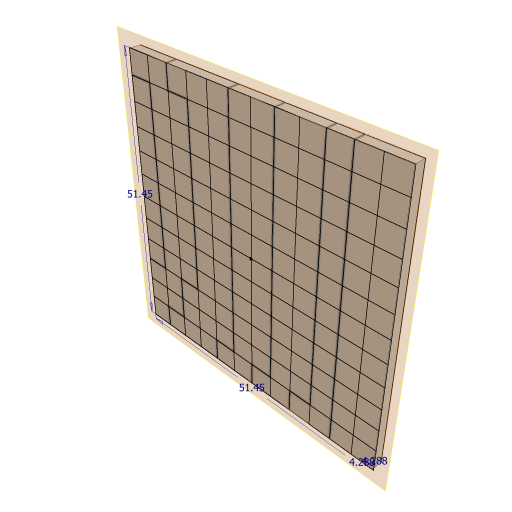
# Autodesk Inventor part: reflector_sketch
Saved by Autodesk Inventor 2023 (Build 270158000, 158)
## iProperties
Created: 2022-08-12
Part Number: reflector_sketch
Material: Generic
Document SubType Name: Modeling
Designer: James
Density: 1 g/cm^3
Appearance: Default
Author: James
Autodesk Inventor part; units mm, degrees
ref_plane "YZ Plane" through (0, 0, 0) normal (1, 0, 0) x (0, 1, 0)
ref_plane "XZ Plane" through (0, 0, 0) normal (0, 1, 0) x (-1, 0, 0)
sketch "construction_sketch" plane through (0, 0, 0) normal (0, 0, 1) x (1, 0, 0)
  line L0 (25.725, 25.725) -> (-25.725, 25.725) construction
  line L1 (-25.725, 25.725) -> (-25.725, -25.725) construction
  line L2 (-25.725, -25.725) -> (25.725, -25.725) construction
  line L3 (25.725, -25.725) -> (25.725, 25.725) construction
  line L4 (25.725, -25.725) -> (17.15, -25.725) construction
  line L5 (17.15, -25.725) -> (17.15, 25.725) construction
  line L6 (17.15, 25.725) -> (25.725, 25.725) construction
  line L7 (25.725, 25.725) -> (25.725, -25.725) construction
  line L8 (17.15, 25.725) -> (12.8625, 25.725) construction
  line L9 (12.8625, 25.725) -> (12.8625, -21.4375) construction
  line L10 (17.15, -25.725) -> (17.15, 25.725) construction
  line L11 (17.15, -25.725) -> (8.575, -25.725) construction
  line L12 (8.575, -25.725) -> (8.575, -21.4375) construction
  line L13 (8.575, -21.4375) -> (12.8625, -21.4375) construction
  line L14 (12.8625, 25.725) -> (4.2875, 25.725) construction
  line L15 (4.2875, 25.725) -> (4.2875, -21.4375) construction
  line L16 (8.575, -21.4375) -> (12.8625, -21.4375) construction
  line L17 (12.8625, -21.4375) -> (12.8625, 25.725) construction
  line L18 (8.575, -25.725) -> (0, -25.725) construction
  line L19 (0, -25.725) -> (0, -21.4375) construction
  line L20 (0, -21.4375) -> (4.2875, -21.4375) construction
  line L21 (8.575, -21.4375) -> (8.575, -25.725) construction
  line L22 (4.2875, 25.725) -> (4.2875, -21.4375) construction
  line L23 (0, -25.725) -> (0, -21.4375) construction
  line L24 (0, -21.4375) -> (4.2875, -21.4375) construction
  line L25 (4.2875, 25.725) -> (-4.2875, 25.725) construction
  line L26 (-4.2875, 25.725) -> (-4.2875, -21.4375) construction
  line L27 (0, -21.4375) -> (4.2875, -21.4375) construction
  line L28 (4.2875, -21.4375) -> (4.2875, 25.725) construction
  line L29 (0, -25.725) -> (-8.575, -25.725) construction
  line L30 (-8.575, -25.725) -> (-8.575, -21.4375) construction
  line L31 (-8.575, -21.4375) -> (-4.2875, -21.4375) construction
  line L32 (0, -21.4375) -> (0, -25.725) construction
  line L33 (-4.2875, 25.725) -> (-17.15, 25.725) construction
  line L34 (-17.15, 25.725) -> (-17.15, 21.4375) construction
  line L35 (-17.15, 21.4375) -> (-12.8625, 21.4375) construction
  line L36 (-4.2875, 21.4375) -> (-4.2875, 25.725) construction
  line L37 (-4.2875, -21.4375) -> (-8.575, -21.4375) construction
  line L38 (-17.15, -21.4375) -> (-17.15, -12.8625) construction
  line L39 (-17.15, -12.8625) -> (-12.8625, -12.8625) construction
  line L40 (-4.2875, -12.8625) -> (-4.2875, -21.4375) construction
  line L41 (-12.8625, -12.8625) -> (-12.8625, 21.4375) construction
  line L42 (-4.2875, 21.4375) -> (-4.2875, -12.8625) construction
  line L43 (-17.15, -21.4375) -> (-21.4375, -21.4375) construction
  line L44 (-21.4375, -21.4375) -> (-21.4375, -25.725) construction
  line L45 (-21.4375, -25.725) -> (-8.575, -25.725) construction
  line L46 (-8.575, -25.725) -> (-8.575, -21.4375) construction
  line L47 (-25.725, -12.8625) -> (-21.4375, -12.8625) construction
  line L48 (-21.4375, -12.8625) -> (-21.4375, 21.4375) construction
  line L49 (-21.4375, 21.4375) -> (-25.725, 21.4375) construction
  line L50 (-25.725, 21.4375) -> (-25.725, -12.8625) construction
  point P0 (0, 0)
  constraints: 102 end point, 23 parallel, 12 horizontal, 12 perpendicular, 6 point on line
sketch "construction_sketch_2" plane through (0, 0, 0) normal (0, 0, 1) x (1, 0, 0)
  line L0 (-17.15, -12.8625) -> (-12.8625, -12.8625) construction
  line L1 (25.625, 25.625) -> (25.625, -25.625) construction
  line L2 (25.625, -25.625) -> (17.25, -25.625) construction
  line L3 (17.25, -25.625) -> (17.25, 25.625) construction
  line L4 (-8.475, -25.625) -> (-8.475, -21.5375) construction
  line L5 (-8.475, -21.5375) -> (-4.1875, -21.5375) construction
  line L6 (-4.1875, -21.5375) -> (-4.1875, 25.625) construction
  line L7 (-4.1875, 25.625) -> (4.1875, 25.625) construction
  line L8 (4.1875, 25.625) -> (4.1875, -21.3375) construction
  line L9 (4.1875, -21.3375) -> (-0.1, -21.3375) construction
  line L10 (-0.1, -21.3375) -> (-0.1, -25.625) construction
  line L11 (-0.1, -25.625) -> (-8.475, -25.625) construction
  line L12 (17.25, 25.625) -> (25.625, 25.625) construction
  line L13 (4.388, 25.625) -> (12.7625, 25.625) construction
  line L14 (12.7625, 25.625) -> (12.7625, -21.3375) construction
  line L15 (12.7625, -21.3375) -> (8.475, -21.3375) construction
  line L16 (8.475, -21.3375) -> (8.475, -25.625) construction
  line L17 (8.475, -25.625) -> (0.1, -25.625) construction
  line L18 (0.1, -25.625) -> (0.1, -21.5375) construction
  line L19 (0.1, -21.5375) -> (4.388, -21.5375) construction
  line L20 (4.388, 25.625) -> (4.388, -21.5375) construction
  line L21 (17.05, -25.625) -> (17.05, 25.625) construction
  line L22 (17.05, -25.625) -> (8.675, -25.625) construction
  line L23 (8.675, -25.625) -> (8.675, -21.5375) construction
  line L24 (17.05, 25.625) -> (12.9625, 25.625) construction
  line L25 (12.9625, 25.625) -> (12.9625, -21.5375) construction
  line L26 (12.9625, -21.5375) -> (8.675, -21.5375) construction
  line L27 (-21.3375, -25.625) -> (-8.675, -25.625) construction
  line L28 (-17.0505, -21.5375) -> (-21.3375, -21.5375) construction
  line L29 (-21.3375, -21.5375) -> (-21.3375, -25.625) construction
  line L30 (-4.3875, -21.3375) -> (-8.675, -21.3375) construction
  line L31 (-4.3875, -21.3375) -> (-4.3875, 25.625) construction
  line L32 (-8.675, -25.625) -> (-8.675, -21.3375) construction
  line L33 (-4.3875, 25.625) -> (-17.0505, 25.625) construction
  line L34 (-17.0505, 25.625) -> (-17.0505, 21.537) construction
  line L35 (-17.0505, 21.537) -> (-12.7625, 21.537) construction
  line L36 (-17.0505, -21.5375) -> (-17.0505, -12.9625) construction
  line L37 (-17.0505, -12.9625) -> (-12.7625, -12.9625) construction
  line L38 (-12.7625, -12.9625) -> (-12.7625, 21.537) construction
  line L39 (-21.5375, -12.7625) -> (-25.625, -12.7625) construction
  line L40 (-25.625, -12.7625) -> (-25.625, 21.3375) construction
  line L41 (-25.625, 21.3375) -> (-21.5375, 21.3375) construction
  line L42 (-21.5375, 21.3375) -> (-21.5375, -12.7625) construction
  line L43 (-25.625, 21.5375) -> (-25.625, 25.625) construction
  line L44 (-25.625, 25.625) -> (-17.25, 25.625) construction
  line L45 (-17.25, 25.625) -> (-17.25, 21.3375) construction
  line L46 (-17.25, 21.3375) -> (-12.9625, 21.3375) construction
  line L47 (-12.9625, 21.3375) -> (-12.9625, -12.7625) construction
  line L48 (-12.9625, -12.7625) -> (-17.25, -12.7625) construction
  line L49 (-17.25, -12.7625) -> (-17.25, -21.3375) construction
  line L50 (-17.25, -21.3375) -> (-21.5375, -21.3375) construction
  line L51 (-21.5375, -21.3375) -> (-21.5375, -25.625) construction
  line L52 (-25.625, -12.9625) -> (-25.625, -25.625) construction
  line L53 (-25.625, -25.625) -> (-21.5375, -25.625) construction
  line L54 (-21.3375, -12.9625) -> (-25.625, -12.9625) construction
  line L55 (-25.625, 21.5375) -> (-21.3375, 21.5375) construction
  line L56 (-21.3375, 21.5375) -> (-21.3375, -12.9625) construction
  point P0 (0, 0)
  constraints: 114 end point, 18 perpendicular, 8 parallel, 2 horizontal, 1 point on line, 1 vertical
sketch "brick_sketch_0.1mm tolerance" plane through (0, 0, 0) normal (0, 0, 1) x (1, 0, 0)
  line L0 (-17.15, -12.8625) -> (-12.8625, -12.8625) construction
  line L1 (25.625, 25.625) -> (25.625, -25.625)
  line L2 (25.625, -25.625) -> (17.25, -25.625)
  line L3 (17.25, -25.625) -> (17.25, 25.625)
  line L4 (-8.475, -25.625) -> (-8.475, -21.5375)
  line L5 (-8.475, -21.5375) -> (-4.1875, -21.5375)
  line L6 (-4.1875, -21.5375) -> (-4.1875, 25.625)
  line L7 (-4.1875, 25.625) -> (4.1875, 25.625)
  line L8 (4.1875, 25.625) -> (4.1875, -21.3375)
  line L9 (4.1875, -21.3375) -> (-0.1, -21.3375)
  line L10 (-0.1, -21.3375) -> (-0.1, -25.625)
  line L11 (-0.1, -25.625) -> (-8.475, -25.625)
  line L12 (17.25, 25.625) -> (25.625, 25.625)
  line L13 (4.388, 25.625) -> (12.7625, 25.625)
  line L14 (12.7625, 25.625) -> (12.7625, -21.3375)
  line L15 (12.7625, -21.3375) -> (8.475, -21.3375)
  line L16 (8.475, -21.3375) -> (8.475, -25.625)
  line L17 (8.475, -25.625) -> (0.1, -25.625)
  line L18 (0.1, -25.625) -> (0.1, -21.5375)
  line L19 (0.1, -21.5375) -> (4.388, -21.5375)
  line L20 (4.388, 25.625) -> (4.388, -21.5375)
  line L21 (17.05, -25.625) -> (17.05, 25.625)
  line L22 (17.05, -25.625) -> (8.675, -25.625)
  line L23 (8.675, -25.625) -> (8.675, -21.5375)
  line L24 (17.05, 25.625) -> (12.9625, 25.625)
  line L25 (12.9625, 25.625) -> (12.9625, -21.5375)
  line L26 (12.9625, -21.5375) -> (8.675, -21.5375)
  line L27 (-21.3375, -25.625) -> (-8.675, -25.625)
  line L28 (-17.0505, -21.5375) -> (-21.3375, -21.5375)
  line L29 (-21.3375, -21.5375) -> (-21.3375, -25.625)
  line L30 (-4.3875, -21.3375) -> (-8.675, -21.3375)
  line L31 (-4.3875, -21.3375) -> (-4.3875, 25.625)
  line L32 (-8.675, -25.625) -> (-8.675, -21.3375)
  line L33 (-4.3875, 25.625) -> (-17.0505, 25.625)
  line L34 (-17.0505, 25.625) -> (-17.0505, 21.537)
  line L35 (-17.0505, 21.537) -> (-12.7625, 21.537)
  line L36 (-17.0505, -21.5375) -> (-17.0505, -12.9625)
  line L37 (-17.0505, -12.9625) -> (-12.7625, -12.9625)
  line L38 (-12.7625, -12.9625) -> (-12.7625, 21.537)
  line L39 (-21.5375, -12.7625) -> (-25.625, -12.7625)
  line L40 (-25.625, -12.7625) -> (-25.625, 21.3375)
  line L41 (-25.625, 21.3375) -> (-21.5375, 21.3375)
  line L42 (-21.5375, 21.3375) -> (-21.5375, -12.7625)
  line L43 (-25.625, 21.5375) -> (-25.625, 25.625)
  line L44 (-25.625, 25.625) -> (-17.25, 25.625)
  line L45 (-17.25, 25.625) -> (-17.25, 21.3375)
  line L46 (-17.25, 21.3375) -> (-12.9625, 21.3375)
  line L47 (-12.9625, 21.3375) -> (-12.9625, -12.7625)
  line L48 (-12.9625, -12.7625) -> (-17.25, -12.7625)
  line L49 (-17.25, -12.7625) -> (-17.25, -21.3375)
  line L50 (-17.25, -21.3375) -> (-21.5375, -21.3375)
  line L51 (-21.5375, -21.3375) -> (-21.5375, -25.625)
  line L52 (-25.625, -12.9625) -> (-25.625, -25.625)
  line L53 (-25.625, -25.625) -> (-21.5375, -25.625)
  line L54 (-21.3375, -12.9625) -> (-25.625, -12.9625)
  line L55 (-25.625, 21.5375) -> (-21.3375, 21.5375)
  line L56 (-21.3375, 21.5375) -> (-21.3375, -12.9625)
  point P0 (0, 0)
  point P1 (0, 0)
  constraints: 114 end point, 18 perpendicular, 8 parallel, 2 horizontal, 1 point on line, 1 vertical
ref_plane "Work Plane1" through (0, 0, 2) normal (0, 0, 1) x (1, 0, 0)
sketch "Sketch4" plane through (0, 0, 2) normal (0, 0, 1) x (1, 0, 0)
  line L0 (25.725, 25.725) -> (-25.725, 25.725) construction
  line L1 (-25.725, 25.725) -> (-25.725, -25.725) construction
  line L2 (-25.725, -25.725) -> (25.725, -25.725) construction
  line L3 (25.725, -25.725) -> (25.725, 25.725) construction
  line L4 (25.725, -25.725) -> (21.4375, -25.725)
  line L5 (21.4375, -25.725) -> (21.4375, -21.4375)
  line L6 (21.4375, -21.4375) -> (25.725, -21.4375)
  line L7 (25.725, -21.4375) -> (25.725, -25.725)
  line L8 (21.4375, -25.725) -> (17.15, -25.725)
  line L9 (17.15, -25.725) -> (17.15, -21.4375)
  line L10 (17.15, -21.4375) -> (21.4375, -21.4375)
  line L11 (21.4375, -21.4375) -> (21.4375, -25.725)
  line L12 (17.15, -25.725) -> (12.8625, -25.725)
  line L13 (12.8625, -25.725) -> (12.8625, -21.4375)
  line L14 (12.8625, -21.4375) -> (17.15, -21.4375)
  line L15 (17.15, -21.4375) -> (17.15, -25.725)
  line L16 (12.8625, -25.725) -> (8.575, -25.725)
  line L17 (8.575, -25.725) -> (8.575, -21.4375)
  line L18 (8.575, -21.4375) -> (12.8625, -21.4375)
  line L19 (12.8625, -21.4375) -> (12.8625, -25.725)
  line L20 (8.575, -25.725) -> (4.2875, -25.725)
  line L21 (4.2875, -25.725) -> (4.2875, -21.4375)
  line L22 (4.2875, -21.4375) -> (8.575, -21.4375)
  line L23 (8.575, -21.4375) -> (8.575, -25.725)
  line L24 (4.2875, -25.725) -> (0, -25.725)
  line L25 (0, -25.725) -> (0, -21.4375)
  line L26 (0, -21.4375) -> (4.2875, -21.4375)
  line L27 (4.2875, -21.4375) -> (4.2875, -25.725)
  line L28 (0, -25.725) -> (-4.2875, -25.725)
  line L29 (-4.2875, -25.725) -> (-4.2875, -21.4375)
  line L30 (-4.2875, -21.4375) -> (0, -21.4375)
  line L31 (0, -21.4375) -> (0, -25.725)
  line L32 (-4.2875, -25.725) -> (-8.575, -25.725)
  line L33 (-8.575, -25.725) -> (-8.575, -21.4375)
  line L34 (-8.575, -21.4375) -> (-4.2875, -21.4375)
  line L35 (-4.2875, -21.4375) -> (-4.2875, -25.725)
  line L36 (-8.575, -25.725) -> (-12.8625, -25.725)
  line L37 (-12.8625, -25.725) -> (-12.8625, -21.4375)
  line L38 (-12.8625, -21.4375) -> (-8.575, -21.4375)
  line L39 (-8.575, -21.4375) -> (-8.575, -25.725)
  line L40 (-12.8625, -25.725) -> (-17.15, -25.725)
  line L41 (-17.15, -25.725) -> (-17.15, -21.4375)
  line L42 (-17.15, -21.4375) -> (-12.8625, -21.4375)
  line L43 (-12.8625, -21.4375) -> (-12.8625, -25.725)
  line L44 (-17.15, -25.725) -> (-21.4375, -25.725)
  line L45 (-21.4375, -25.725) -> (-21.4375, -21.4375)
  line L46 (-21.4375, -21.4375) -> (-17.15, -21.4375)
  line L47 (-17.15, -21.4375) -> (-17.15, -25.725)
  line L48 (-21.4375, -25.725) -> (-25.725, -25.725)
  line L49 (-25.725, -25.725) -> (-25.725, -21.4375)
  line L50 (-25.725, -21.4375) -> (-21.4375, -21.4375)
  line L51 (-21.4375, -21.4375) -> (-21.4375, -25.725)
  line L52 (25.725, -21.4375) -> (21.4375, -21.4375)
  line L53 (21.4375, -21.4375) -> (21.4375, -17.15)
  line L54 (21.4375, -17.15) -> (25.725, -17.15)
  line L55 (25.725, -17.15) -> (25.725, -21.4375)
  line L56 (21.4375, -21.4375) -> (17.15, -21.4375)
  line L57 (17.15, -21.4375) -> (17.15, -17.15)
  line L58 (17.15, -17.15) -> (21.4375, -17.15)
  line L59 (21.4375, -17.15) -> (21.4375, -21.4375)
  line L60 (17.15, -21.4375) -> (12.8625, -21.4375)
  line L61 (12.8625, -21.4375) -> (12.8625, -17.15)
  line L62 (12.8625, -17.15) -> (17.15, -17.15)
  line L63 (17.15, -17.15) -> (17.15, -21.4375)
  line L64 (12.8625, -21.4375) -> (8.575, -21.4375)
  line L65 (8.575, -21.4375) -> (8.575, -17.15)
  line L66 (8.575, -17.15) -> (12.8625, -17.15)
  line L67 (12.8625, -17.15) -> (12.8625, -21.4375)
  line L68 (8.575, -21.4375) -> (4.2875, -21.4375)
  line L69 (4.2875, -21.4375) -> (4.2875, -17.15)
  line L70 (4.2875, -17.15) -> (8.575, -17.15)
  line L71 (8.575, -17.15) -> (8.575, -21.4375)
  line L72 (4.2875, -21.4375) -> (0, -21.4375)
  line L73 (0, -21.4375) -> (0, -17.15)
  line L74 (0, -17.15) -> (4.2875, -17.15)
  line L75 (4.2875, -17.15) -> (4.2875, -21.4375)
  line L76 (0, -21.4375) -> (-4.2875, -21.4375)
  line L77 (-4.2875, -21.4375) -> (-4.2875, -17.15)
  line L78 (-4.2875, -17.15) -> (0, -17.15)
  line L79 (0, -17.15) -> (0, -21.4375)
  line L80 (-4.2875, -21.4375) -> (-8.575, -21.4375)
  line L81 (-8.575, -21.4375) -> (-8.575, -17.15)
  line L82 (-8.575, -17.15) -> (-4.2875, -17.15)
  line L83 (-4.2875, -17.15) -> (-4.2875, -21.4375)
  line L84 (-8.575, -21.4375) -> (-12.8625, -21.4375)
  line L85 (-12.8625, -21.4375) -> (-12.8625, -17.15)
  line L86 (-12.8625, -17.15) -> (-8.575, -17.15)
  line L87 (-8.575, -17.15) -> (-8.575, -21.4375)
  line L88 (-12.8625, -21.4375) -> (-17.15, -21.4375)
  line L89 (-17.15, -21.4375) -> (-17.15, -17.15)
  line L90 (-17.15, -17.15) -> (-12.8625, -17.15)
  line L91 (-12.8625, -17.15) -> (-12.8625, -21.4375)
  line L92 (-17.15, -21.4375) -> (-21.4375, -21.4375)
  line L93 (-21.4375, -21.4375) -> (-21.4375, -17.15)
  line L94 (-21.4375, -17.15) -> (-17.15, -17.15)
  line L95 (-17.15, -17.15) -> (-17.15, -21.4375)
  line L96 (-21.4375, -21.4375) -> (-25.725, -21.4375)
  line L97 (-25.725, -21.4375) -> (-25.725, -17.15)
  line L98 (-25.725, -17.15) -> (-21.4375, -17.15)
  line L99 (-21.4375, -17.15) -> (-21.4375, -21.4375)
  line L100 (25.725, -17.15) -> (21.4375, -17.15)
  line L101 (21.4375, -17.15) -> (21.4375, -12.8625)
  line L102 (21.4375, -12.8625) -> (25.725, -12.8625)
  line L103 (25.725, -12.8625) -> (25.725, -17.15)
  line L104 (21.4375, -17.15) -> (17.15, -17.15)
  line L105 (17.15, -17.15) -> (17.15, -12.8625)
  line L106 (17.15, -12.8625) -> (21.4375, -12.8625)
  line L107 (21.4375, -12.8625) -> (21.4375, -17.15)
  line L108 (17.15, -17.15) -> (12.8625, -17.15)
  line L109 (12.8625, -17.15) -> (12.8625, -12.8625)
  line L110 (12.8625, -12.8625) -> (17.15, -12.8625)
  line L111 (17.15, -12.8625) -> (17.15, -17.15)
  line L112 (12.8625, -17.15) -> (8.575, -17.15)
  line L113 (8.575, -17.15) -> (8.575, -12.8625)
  line L114 (8.575, -12.8625) -> (12.8625, -12.8625)
  line L115 (12.8625, -12.8625) -> (12.8625, -17.15)
  line L116 (8.575, -17.15) -> (4.2875, -17.15)
  line L117 (4.2875, -17.15) -> (4.2875, -12.8625)
  line L118 (4.2875, -12.8625) -> (8.575, -12.8625)
  line L119 (8.575, -12.8625) -> (8.575, -17.15)
  line L120 (4.2875, -17.15) -> (0, -17.15)
  line L121 (0, -17.15) -> (0, -12.8625)
  line L122 (0, -12.8625) -> (4.2875, -12.8625)
  line L123 (4.2875, -12.8625) -> (4.2875, -17.15)
  line L124 (0, -17.15) -> (-4.2875, -17.15)
  line L125 (-4.2875, -17.15) -> (-4.2875, -12.8625)
  line L126 (-4.2875, -12.8625) -> (0, -12.8625)
  line L127 (0, -12.8625) -> (0, -17.15)
  line L128 (-4.2875, -17.15) -> (-8.575, -17.15)
  line L129 (-8.575, -17.15) -> (-8.575, -12.8625)
  line L130 (-8.575, -12.8625) -> (-4.2875, -12.8625)
  line L131 (-4.2875, -12.8625) -> (-4.2875, -17.15)
  line L132 (-8.575, -17.15) -> (-12.8625, -17.15)
  line L133 (-12.8625, -17.15) -> (-12.8625, -12.8625)
  line L134 (-12.8625, -12.8625) -> (-8.575, -12.8625)
  line L135 (-8.575, -12.8625) -> (-8.575, -17.15)
  line L136 (-12.8625, -17.15) -> (-17.15, -17.15)
  line L137 (-17.15, -17.15) -> (-17.15, -12.8625)
  line L138 (-17.15, -12.8625) -> (-12.8625, -12.8625)
  line L139 (-12.8625, -12.8625) -> (-12.8625, -17.15)
  line L140 (-17.15, -17.15) -> (-21.4375, -17.15)
  line L141 (-21.4375, -17.15) -> (-21.4375, -12.8625)
  line L142 (-21.4375, -12.8625) -> (-17.15, -12.8625)
  line L143 (-17.15, -12.8625) -> (-17.15, -17.15)
  line L144 (-21.4375, -17.15) -> (-25.725, -17.15)
  line L145 (-25.725, -17.15) -> (-25.725, -12.8625)
  line L146 (-25.725, -12.8625) -> (-21.4375, -12.8625)
  line L147 (-21.4375, -12.8625) -> (-21.4375, -17.15)
  line L148 (25.725, -12.8625) -> (21.4375, -12.8625)
  line L149 (21.4375, -12.8625) -> (21.4375, -8.575)
  line L150 (21.4375, -8.575) -> (25.725, -8.575)
  line L151 (25.725, -8.575) -> (25.725, -12.8625)
  line L152 (21.4375, -12.8625) -> (17.15, -12.8625)
  line L153 (17.15, -12.8625) -> (17.15, -8.575)
  line L154 (17.15, -8.575) -> (21.4375, -8.575)
  line L155 (21.4375, -8.575) -> (21.4375, -12.8625)
  line L156 (17.15, -12.8625) -> (12.8625, -12.8625)
  line L157 (12.8625, -12.8625) -> (12.8625, -8.575)
  line L158 (12.8625, -8.575) -> (17.15, -8.575)
  line L159 (17.15, -8.575) -> (17.15, -12.8625)
  line L160 (12.8625, -12.8625) -> (8.575, -12.8625)
  line L161 (8.575, -12.8625) -> (8.575, -8.575)
  line L162 (8.575, -8.575) -> (12.8625, -8.575)
  line L163 (12.8625, -8.575) -> (12.8625, -12.8625)
  line L164 (8.575, -12.8625) -> (4.2875, -12.8625)
  line L165 (4.2875, -12.8625) -> (4.2875, -8.575)
  line L166 (4.2875, -8.575) -> (8.575, -8.575)
  line L167 (8.575, -8.575) -> (8.575, -12.8625)
  line L168 (4.2875, -12.8625) -> (0, -12.8625)
  line L169 (0, -12.8625) -> (0, -8.575)
  line L170 (0, -8.575) -> (4.2875, -8.575)
  line L171 (4.2875, -8.575) -> (4.2875, -12.8625)
  line L172 (0, -12.8625) -> (-4.2875, -12.8625)
  line L173 (-4.2875, -12.8625) -> (-4.2875, -8.575)
  line L174 (-4.2875, -8.575) -> (0, -8.575)
  line L175 (0, -8.575) -> (0, -12.8625)
  line L176 (-4.2875, -12.8625) -> (-8.575, -12.8625)
  line L177 (-8.575, -12.8625) -> (-8.575, -8.575)
  line L178 (-8.575, -8.575) -> (-4.2875, -8.575)
  line L179 (-4.2875, -8.575) -> (-4.2875, -12.8625)
  line L180 (-8.575, -12.8625) -> (-12.8625, -12.8625)
  line L181 (-12.8625, -12.8625) -> (-12.8625, -8.575)
  line L182 (-12.8625, -8.575) -> (-8.575, -8.575)
  line L183 (-8.575, -8.575) -> (-8.575, -12.8625)
  line L184 (-12.8625, -12.8625) -> (-17.15, -12.8625)
  line L185 (-17.15, -12.8625) -> (-17.15, -8.575)
  line L186 (-17.15, -8.575) -> (-12.8625, -8.575)
  line L187 (-12.8625, -8.575) -> (-12.8625, -12.8625)
  line L188 (-17.15, -12.8625) -> (-21.4375, -12.8625)
  line L189 (-21.4375, -12.8625) -> (-21.4375, -8.575)
  line L190 (-21.4375, -8.575) -> (-17.15, -8.575)
  line L191 (-17.15, -8.575) -> (-17.15, -12.8625)
  line L192 (-21.4375, -12.8625) -> (-25.725, -12.8625)
  line L193 (-25.725, -12.8625) -> (-25.725, -8.575)
  line L194 (-25.725, -8.575) -> (-21.4375, -8.575)
  line L195 (-21.4375, -8.575) -> (-21.4375, -12.8625)
  line L196 (25.725, -8.575) -> (21.4375, -8.575)
  line L197 (21.4375, -8.575) -> (21.4375, -4.2875)
  line L198 (21.4375, -4.2875) -> (25.725, -4.2875)
  line L199 (25.725, -4.2875) -> (25.725, -8.575)
  line L200 (21.4375, -8.575) -> (17.15, -8.575)
  line L201 (17.15, -8.575) -> (17.15, -4.2875)
  line L202 (17.15, -4.2875) -> (21.4375, -4.2875)
  line L203 (21.4375, -4.2875) -> (21.4375, -8.575)
  line L204 (17.15, -8.575) -> (12.8625, -8.575)
  line L205 (12.8625, -8.575) -> (12.8625, -4.2875)
  line L206 (12.8625, -4.2875) -> (17.15, -4.2875)
  line L207 (17.15, -4.2875) -> (17.15, -8.575)
  line L208 (12.8625, -8.575) -> (8.575, -8.575)
  line L209 (8.575, -8.575) -> (8.575, -4.2875)
  line L210 (8.575, -4.2875) -> (12.8625, -4.2875)
  line L211 (12.8625, -4.2875) -> (12.8625, -8.575)
  line L212 (8.575, -8.575) -> (4.2875, -8.575)
  line L213 (4.2875, -8.575) -> (4.2875, -4.2875)
  line L214 (4.2875, -4.2875) -> (8.575, -4.2875)
  line L215 (8.575, -4.2875) -> (8.575, -8.575)
  line L216 (4.2875, -8.575) -> (0, -8.575)
  line L217 (0, -8.575) -> (0, -4.2875)
  line L218 (0, -4.2875) -> (4.2875, -4.2875)
  line L219 (4.2875, -4.2875) -> (4.2875, -8.575)
  line L220 (0, -8.575) -> (-4.2875, -8.575)
  line L221 (-4.2875, -8.575) -> (-4.2875, -4.2875)
  line L222 (-4.2875, -4.2875) -> (0, -4.2875)
  line L223 (0, -4.2875) -> (0, -8.575)
  line L224 (-4.2875, -8.575) -> (-8.575, -8.575)
  line L225 (-8.575, -8.575) -> (-8.575, -4.2875)
  line L226 (-8.575, -4.2875) -> (-4.2875, -4.2875)
  line L227 (-4.2875, -4.2875) -> (-4.2875, -8.575)
  line L228 (-8.575, -8.575) -> (-12.8625, -8.575)
  line L229 (-12.8625, -8.575) -> (-12.8625, -4.2875)
  line L230 (-12.8625, -4.2875) -> (-8.575, -4.2875)
  line L231 (-8.575, -4.2875) -> (-8.575, -8.575)
  line L232 (-12.8625, -8.575) -> (-17.15, -8.575)
  line L233 (-17.15, -8.575) -> (-17.15, -4.2875)
  line L234 (-17.15, -4.2875) -> (-12.8625, -4.2875)
  line L235 (-12.8625, -4.2875) -> (-12.8625, -8.575)
  line L236 (-17.15, -8.575) -> (-21.4375, -8.575)
  line L237 (-21.4375, -8.575) -> (-21.4375, -4.2875)
  line L238 (-21.4375, -4.2875) -> (-17.15, -4.2875)
  line L239 (-17.15, -4.2875) -> (-17.15, -8.575)
  line L240 (-21.4375, -8.575) -> (-25.725, -8.575)
  line L241 (-25.725, -8.575) -> (-25.725, -4.2875)
  line L242 (-25.725, -4.2875) -> (-21.4375, -4.2875)
  line L243 (-21.4375, -4.2875) -> (-21.4375, -8.575)
  line L244 (25.725, -4.2875) -> (21.4375, -4.2875)
  line L245 (21.4375, -4.2875) -> (21.4375, 0)
  line L246 (21.4375, 0) -> (25.725, 0)
  line L247 (25.725, 0) -> (25.725, -4.2875)
  line L248 (21.4375, -4.2875) -> (17.15, -4.2875)
  line L249 (17.15, -4.2875) -> (17.15, 0)
  line L250 (17.15, 0) -> (21.4375, 0)
  line L251 (21.4375, 0) -> (21.4375, -4.2875)
  line L252 (17.15, -4.2875) -> (12.8625, -4.2875)
  line L253 (12.8625, -4.2875) -> (12.8625, 0)
  line L254 (12.8625, 0) -> (17.15, 0)
  line L255 (17.15, 0) -> (17.15, -4.2875)
  line L256 (12.8625, -4.2875) -> (8.575, -4.2875)
  line L257 (8.575, -4.2875) -> (8.575, 0)
  line L258 (8.575, 0) -> (12.8625, 0)
  line L259 (12.8625, 0) -> (12.8625, -4.2875)
  line L260 (8.575, -4.2875) -> (4.2875, -4.2875)
  line L261 (4.2875, -4.2875) -> (4.2875, 0)
  line L262 (4.2875, 0) -> (8.575, 0)
  line L263 (8.575, 0) -> (8.575, -4.2875)
  line L264 (4.2875, -4.2875) -> (0, -4.2875)
  line L265 (0, -4.2875) -> (0, 0)
  line L266 (0, 0) -> (4.2875, 0)
  line L267 (4.2875, 0) -> (4.2875, -4.2875)
  line L268 (0, -4.2875) -> (-4.2875, -4.2875)
  line L269 (-4.2875, -4.2875) -> (-4.2875, 0)
  line L270 (-4.2875, 0) -> (0, 0)
  line L271 (0, 0) -> (0, -4.2875)
  line L272 (-4.2875, -4.2875) -> (-8.575, -4.2875)
  line L273 (-8.575, -4.2875) -> (-8.575, 0)
  line L274 (-8.575, 0) -> (-4.2875, 0)
  line L275 (-4.2875, 0) -> (-4.2875, -4.2875)
  line L276 (-8.575, -4.2875) -> (-12.8625, -4.2875)
  line L277 (-12.8625, -4.2875) -> (-12.8625, 0)
  line L278 (-12.8625, 0) -> (-8.575, 0)
  line L279 (-8.575, 0) -> (-8.575, -4.2875)
  line L280 (-12.8625, -4.2875) -> (-17.15, -4.2875)
  line L281 (-17.15, -4.2875) -> (-17.15, 0)
  line L282 (-17.15, 0) -> (-12.8625, 0)
  line L283 (-12.8625, 0) -> (-12.8625, -4.2875)
  line L284 (-17.15, -4.2875) -> (-21.4375, -4.2875)
  line L285 (-21.4375, -4.2875) -> (-21.4375, 0)
  line L286 (-21.4375, 0) -> (-17.15, 0)
  line L287 (-17.15, 0) -> (-17.15, -4.2875)
  line L288 (-21.4375, -4.2875) -> (-25.725, -4.2875)
  line L289 (-25.725, -4.2875) -> (-25.725, 0)
  line L290 (-25.725, 0) -> (-21.4375, 0)
  line L291 (-21.4375, 0) -> (-21.4375, -4.2875)
  line L292 (25.725, 0) -> (21.4375, 0)
  line L293 (21.4375, 0) -> (21.4375, 4.2875)
  line L294 (21.4375, 4.2875) -> (25.725, 4.2875)
  line L295 (25.725, 4.2875) -> (25.725, 0)
  line L296 (21.4375, 0) -> (17.15, 0)
  line L297 (17.15, 0) -> (17.15, 4.2875)
  line L298 (17.15, 4.2875) -> (21.4375, 4.2875)
  line L299 (21.4375, 4.2875) -> (21.4375, 0)
  line L300 (17.15, 0) -> (12.8625, 0)
  line L301 (12.8625, 0) -> (12.8625, 4.2875)
  line L302 (12.8625, 4.2875) -> (17.15, 4.2875)
  line L303 (17.15, 4.2875) -> (17.15, 0)
  line L304 (12.8625, 0) -> (8.575, 0)
  line L305 (8.575, 0) -> (8.575, 4.2875)
  line L306 (8.575, 4.2875) -> (12.8625, 4.2875)
  line L307 (12.8625, 4.2875) -> (12.8625, 0)
  line L308 (8.575, 0) -> (4.2875, 0)
  line L309 (4.2875, 0) -> (4.2875, 4.2875)
  line L310 (4.2875, 4.2875) -> (8.575, 4.2875)
  line L311 (8.575, 4.2875) -> (8.575, 0)
  line L312 (4.2875, 0) -> (0, 0)
  line L313 (0, 0) -> (0, 4.2875)
  line L314 (0, 4.2875) -> (4.2875, 4.2875)
  line L315 (4.2875, 4.2875) -> (4.2875, 0)
  line L316 (0, 0) -> (-4.2875, 0)
  line L317 (-4.2875, 0) -> (-4.2875, 4.2875)
  line L318 (-4.2875, 4.2875) -> (0, 4.2875)
  line L319 (0, 4.2875) -> (0, 0)
  line L320 (-4.2875, 0) -> (-8.575, 0)
  line L321 (-8.575, 0) -> (-8.575, 4.2875)
  line L322 (-8.575, 4.2875) -> (-4.2875, 4.2875)
  line L323 (-4.2875, 4.2875) -> (-4.2875, 0)
  line L324 (-8.575, 0) -> (-12.8625, 0)
  line L325 (-12.8625, 0) -> (-12.8625, 4.2875)
  line L326 (-12.8625, 4.2875) -> (-8.575, 4.2875)
  line L327 (-8.575, 4.2875) -> (-8.575, 0)
  line L328 (-12.8625, 0) -> (-17.15, 0)
  line L329 (-17.15, 0) -> (-17.15, 4.2875)
  line L330 (-17.15, 4.2875) -> (-12.8625, 4.2875)
  line L331 (-12.8625, 4.2875) -> (-12.8625, 0)
  line L332 (-17.15, 0) -> (-21.4375, 0)
  line L333 (-21.4375, 0) -> (-21.4375, 4.2875)
  line L334 (-21.4375, 4.2875) -> (-17.15, 4.2875)
  line L335 (-17.15, 4.2875) -> (-17.15, 0)
  line L336 (-21.4375, 0) -> (-25.725, 0)
  line L337 (-25.725, 0) -> (-25.725, 4.2875)
  line L338 (-25.725, 4.2875) -> (-21.4375, 4.2875)
  line L339 (-21.4375, 4.2875) -> (-21.4375, 0)
  line L340 (25.725, 4.2875) -> (21.4375, 4.2875)
  line L341 (21.4375, 4.2875) -> (21.4375, 8.575)
  line L342 (21.4375, 8.575) -> (25.725, 8.575)
  line L343 (25.725, 8.575) -> (25.725, 4.2875)
  line L344 (21.4375, 4.2875) -> (17.15, 4.2875)
  line L345 (17.15, 4.2875) -> (17.15, 8.575)
  line L346 (17.15, 8.575) -> (21.4375, 8.575)
  line L347 (21.4375, 8.575) -> (21.4375, 4.2875)
  line L348 (17.15, 4.2875) -> (12.8625, 4.2875)
  line L349 (12.8625, 4.2875) -> (12.8625, 8.575)
  line L350 (12.8625, 8.575) -> (17.15, 8.575)
  line L351 (17.15, 8.575) -> (17.15, 4.2875)
  line L352 (12.8625, 4.2875) -> (8.575, 4.2875)
  line L353 (8.575, 4.2875) -> (8.575, 8.575)
  line L354 (8.575, 8.575) -> (12.8625, 8.575)
  line L355 (12.8625, 8.575) -> (12.8625, 4.2875)
  line L356 (8.575, 4.2875) -> (4.2875, 4.2875)
  line L357 (4.2875, 4.2875) -> (4.2875, 8.575)
  line L358 (4.2875, 8.575) -> (8.575, 8.575)
  line L359 (8.575, 8.575) -> (8.575, 4.2875)
  line L360 (4.2875, 4.2875) -> (0, 4.2875)
  line L361 (0, 4.2875) -> (0, 8.575)
  line L362 (0, 8.575) -> (4.2875, 8.575)
  line L363 (4.2875, 8.575) -> (4.2875, 4.2875)
  line L364 (0, 4.2875) -> (-4.2875, 4.2875)
  line L365 (-4.2875, 4.2875) -> (-4.2875, 8.575)
  line L366 (-4.2875, 8.575) -> (0, 8.575)
  line L367 (0, 8.575) -> (0, 4.2875)
  line L368 (-4.2875, 4.2875) -> (-8.575, 4.2875)
  line L369 (-8.575, 4.2875) -> (-8.575, 8.575)
  line L370 (-8.575, 8.575) -> (-4.2875, 8.575)
  line L371 (-4.2875, 8.575) -> (-4.2875, 4.2875)
  line L372 (-8.575, 4.2875) -> (-12.8625, 4.2875)
  line L373 (-12.8625, 4.2875) -> (-12.8625, 8.575)
  line L374 (-12.8625, 8.575) -> (-8.575, 8.575)
  line L375 (-8.575, 8.575) -> (-8.575, 4.2875)
  line L376 (-12.8625, 4.2875) -> (-17.15, 4.2875)
  line L377 (-17.15, 4.2875) -> (-17.15, 8.575)
  line L378 (-17.15, 8.575) -> (-12.8625, 8.575)
  line L379 (-12.8625, 8.575) -> (-12.8625, 4.2875)
  line L380 (-17.15, 4.2875) -> (-21.4375, 4.2875)
  line L381 (-21.4375, 4.2875) -> (-21.4375, 8.575)
  line L382 (-21.4375, 8.575) -> (-17.15, 8.575)
  line L383 (-17.15, 8.575) -> (-17.15, 4.2875)
  line L384 (-21.4375, 4.2875) -> (-25.725, 4.2875)
  line L385 (-25.725, 4.2875) -> (-25.725, 8.575)
  line L386 (-25.725, 8.575) -> (-21.4375, 8.575)
  line L387 (-21.4375, 8.575) -> (-21.4375, 4.2875)
  line L388 (25.725, 8.575) -> (21.4375, 8.575)
  line L389 (21.4375, 8.575) -> (21.4375, 12.8625)
  line L390 (21.4375, 12.8625) -> (25.725, 12.8625)
  line L391 (25.725, 12.8625) -> (25.725, 8.575)
  line L392 (21.4375, 8.575) -> (17.15, 8.575)
  line L393 (17.15, 8.575) -> (17.15, 12.8625)
  line L394 (17.15, 12.8625) -> (21.4375, 12.8625)
  line L395 (21.4375, 12.8625) -> (21.4375, 8.575)
  line L396 (17.15, 8.575) -> (12.8625, 8.575)
  line L397 (12.8625, 8.575) -> (12.8625, 12.8625)
  line L398 (12.8625, 12.8625) -> (17.15, 12.8625)
  line L399 (17.15, 12.8625) -> (17.15, 8.575)
  line L400 (12.8625, 8.575) -> (8.575, 8.575)
  line L401 (8.575, 8.575) -> (8.575, 12.8625)
  line L402 (8.575, 12.8625) -> (12.8625, 12.8625)
  line L403 (12.8625, 12.8625) -> (12.8625, 8.575)
  line L404 (8.575, 8.575) -> (4.2875, 8.575)
  line L405 (4.2875, 8.575) -> (4.2875, 12.8625)
  line L406 (4.2875, 12.8625) -> (8.575, 12.8625)
  line L407 (8.575, 12.8625) -> (8.575, 8.575)
  line L408 (4.2875, 8.575) -> (0, 8.575)
  line L409 (0, 8.575) -> (0, 12.8625)
  line L410 (0, 12.8625) -> (4.2875, 12.8625)
  line L411 (4.2875, 12.8625) -> (4.2875, 8.575)
  line L412 (0, 8.575) -> (-4.2875, 8.575)
  line L413 (-4.2875, 8.575) -> (-4.2875, 12.8625)
  line L414 (-4.2875, 12.8625) -> (0, 12.8625)
  line L415 (0, 12.8625) -> (0, 8.575)
  line L416 (-4.2875, 8.575) -> (-8.575, 8.575)
  line L417 (-8.575, 8.575) -> (-8.575, 12.8625)
  line L418 (-8.575, 12.8625) -> (-4.2875, 12.8625)
  line L419 (-4.2875, 12.8625) -> (-4.2875, 8.575)
  line L420 (-8.575, 8.575) -> (-12.8625, 8.575)
  line L421 (-12.8625, 8.575) -> (-12.8625, 12.8625)
  line L422 (-12.8625, 12.8625) -> (-8.575, 12.8625)
  line L423 (-8.575, 12.8625) -> (-8.575, 8.575)
  line L424 (-12.8625, 8.575) -> (-17.15, 8.575)
  line L425 (-17.15, 8.575) -> (-17.15, 12.8625)
  line L426 (-17.15, 12.8625) -> (-12.8625, 12.8625)
  line L427 (-12.8625, 12.8625) -> (-12.8625, 8.575)
  line L428 (-17.15, 8.575) -> (-21.4375, 8.575)
  line L429 (-21.4375, 8.575) -> (-21.4375, 12.8625)
  line L430 (-21.4375, 12.8625) -> (-17.15, 12.8625)
  line L431 (-17.15, 12.8625) -> (-17.15, 8.575)
  line L432 (-21.4375, 8.575) -> (-25.725, 8.575)
  line L433 (-25.725, 8.575) -> (-25.725, 12.8625)
  line L434 (-25.725, 12.8625) -> (-21.4375, 12.8625)
  line L435 (-21.4375, 12.8625) -> (-21.4375, 8.575)
  line L436 (25.725, 12.8625) -> (21.4375, 12.8625)
  line L437 (21.4375, 12.8625) -> (21.4375, 17.15)
  line L438 (21.4375, 17.15) -> (25.725, 17.15)
  line L439 (25.725, 17.15) -> (25.725, 12.8625)
  line L440 (21.4375, 12.8625) -> (17.15, 12.8625)
  line L441 (17.15, 12.8625) -> (17.15, 17.15)
  line L442 (17.15, 17.15) -> (21.4375, 17.15)
  line L443 (21.4375, 17.15) -> (21.4375, 12.8625)
  line L444 (17.15, 12.8625) -> (12.8625, 12.8625)
  line L445 (12.8625, 12.8625) -> (12.8625, 17.15)
  line L446 (12.8625, 17.15) -> (17.15, 17.15)
  line L447 (17.15, 17.15) -> (17.15, 12.8625)
  line L448 (12.8625, 12.8625) -> (8.575, 12.8625)
  line L449 (8.575, 12.8625) -> (8.575, 17.15)
  line L450 (8.575, 17.15) -> (12.8625, 17.15)
  line L451 (12.8625, 17.15) -> (12.8625, 12.8625)
  line L452 (8.575, 12.8625) -> (4.2875, 12.8625)
  line L453 (4.2875, 12.8625) -> (4.2875, 17.15)
  line L454 (4.2875, 17.15) -> (8.575, 17.15)
  line L455 (8.575, 17.15) -> (8.575, 12.8625)
  line L456 (4.2875, 12.8625) -> (0, 12.8625)
  line L457 (0, 12.8625) -> (0, 17.15)
  line L458 (0, 17.15) -> (4.2875, 17.15)
  line L459 (4.2875, 17.15) -> (4.2875, 12.8625)
  line L460 (0, 12.8625) -> (-4.2875, 12.8625)
  line L461 (-4.2875, 12.8625) -> (-4.2875, 17.15)
  line L462 (-4.2875, 17.15) -> (0, 17.15)
  line L463 (0, 17.15) -> (0, 12.8625)
  line L464 (-4.2875, 12.8625) -> (-8.575, 12.8625)
  line L465 (-8.575, 12.8625) -> (-8.575, 17.15)
  line L466 (-8.575, 17.15) -> (-4.2875, 17.15)
  line L467 (-4.2875, 17.15) -> (-4.2875, 12.8625)
  line L468 (-8.575, 12.8625) -> (-12.8625, 12.8625)
  line L469 (-12.8625, 12.8625) -> (-12.8625, 17.15)
  line L470 (-12.8625, 17.15) -> (-8.575, 17.15)
  line L471 (-8.575, 17.15) -> (-8.575, 12.8625)
  line L472 (-12.8625, 12.8625) -> (-17.15, 12.8625)
  line L473 (-17.15, 12.8625) -> (-17.15, 17.15)
  line L474 (-17.15, 17.15) -> (-12.8625, 17.15)
  line L475 (-12.8625, 17.15) -> (-12.8625, 12.8625)
  line L476 (-17.15, 12.8625) -> (-21.4375, 12.8625)
  line L477 (-21.4375, 12.8625) -> (-21.4375, 17.15)
  line L478 (-21.4375, 17.15) -> (-17.15, 17.15)
  line L479 (-17.15, 17.15) -> (-17.15, 12.8625)
  line L480 (-21.4375, 12.8625) -> (-25.725, 12.8625)
  line L481 (-25.725, 12.8625) -> (-25.725, 17.15)
  line L482 (-25.725, 17.15) -> (-21.4375, 17.15)
  line L483 (-21.4375, 17.15) -> (-21.4375, 12.8625)
  line L484 (25.725, 17.15) -> (21.4375, 17.15)
  line L485 (21.4375, 17.15) -> (21.4375, 21.4375)
  line L486 (21.4375, 21.4375) -> (25.725, 21.4375)
  line L487 (25.725, 21.4375) -> (25.725, 17.15)
  line L488 (21.4375, 17.15) -> (17.15, 17.15)
  line L489 (17.15, 17.15) -> (17.15, 21.4375)
  line L490 (17.15, 21.4375) -> (21.4375, 21.4375)
  line L491 (21.4375, 21.4375) -> (21.4375, 17.15)
  line L492 (17.15, 17.15) -> (12.8625, 17.15)
  line L493 (12.8625, 17.15) -> (12.8625, 21.4375)
  line L494 (12.8625, 21.4375) -> (17.15, 21.4375)
  line L495 (17.15, 21.4375) -> (17.15, 17.15)
  line L496 (12.8625, 17.15) -> (8.575, 17.15)
  line L497 (8.575, 17.15) -> (8.575, 21.4375)
  line L498 (8.575, 21.4375) -> (12.8625, 21.4375)
  line L499 (12.8625, 21.4375) -> (12.8625, 17.15)
  line L500 (8.575, 17.15) -> (4.2875, 17.15)
  line L501 (4.2875, 17.15) -> (4.2875, 21.4375)
  line L502 (4.2875, 21.4375) -> (8.575, 21.4375)
  line L503 (8.575, 21.4375) -> (8.575, 17.15)
  line L504 (4.2875, 17.15) -> (0, 17.15)
  line L505 (0, 17.15) -> (0, 21.4375)
  line L506 (0, 21.4375) -> (4.2875, 21.4375)
  line L507 (4.2875, 21.4375) -> (4.2875, 17.15)
  line L508 (0, 17.15) -> (-4.2875, 17.15)
  line L509 (-4.2875, 17.15) -> (-4.2875, 21.4375)
  line L510 (-4.2875, 21.4375) -> (0, 21.4375)
  line L511 (0, 21.4375) -> (0, 17.15)
  line L512 (-4.2875, 17.15) -> (-8.575, 17.15)
  line L513 (-8.575, 17.15) -> (-8.575, 21.4375)
  line L514 (-8.575, 21.4375) -> (-4.2875, 21.4375)
  line L515 (-4.2875, 21.4375) -> (-4.2875, 17.15)
  line L516 (-8.575, 17.15) -> (-12.8625, 17.15)
  line L517 (-12.8625, 17.15) -> (-12.8625, 21.4375)
  line L518 (-12.8625, 21.4375) -> (-8.575, 21.4375)
  line L519 (-8.575, 21.4375) -> (-8.575, 17.15)
  line L520 (-12.8625, 17.15) -> (-17.15, 17.15)
  line L521 (-17.15, 17.15) -> (-17.15, 21.4375)
  line L522 (-17.15, 21.4375) -> (-12.8625, 21.4375)
  line L523 (-12.8625, 21.4375) -> (-12.8625, 17.15)
  line L524 (-17.15, 17.15) -> (-21.4375, 17.15)
  line L525 (-21.4375, 17.15) -> (-21.4375, 21.4375)
  line L526 (-21.4375, 21.4375) -> (-17.15, 21.4375)
  line L527 (-17.15, 21.4375) -> (-17.15, 17.15)
  line L528 (-21.4375, 17.15) -> (-25.725, 17.15)
  line L529 (-25.725, 17.15) -> (-25.725, 21.4375)
  line L530 (-25.725, 21.4375) -> (-21.4375, 21.4375)
  line L531 (-21.4375, 21.4375) -> (-21.4375, 17.15)
  line L532 (25.725, 21.4375) -> (21.4375, 21.4375)
  line L533 (21.4375, 21.4375) -> (21.4375, 25.725)
  line L534 (21.4375, 25.725) -> (25.725, 25.725)
  line L535 (25.725, 25.725) -> (25.725, 21.4375)
  line L536 (21.4375, 21.4375) -> (17.15, 21.4375)
  line L537 (17.15, 21.4375) -> (17.15, 25.725)
  line L538 (17.15, 25.725) -> (21.4375, 25.725)
  line L539 (21.4375, 25.725) -> (21.4375, 21.4375)
  line L540 (17.15, 21.4375) -> (12.8625, 21.4375)
  line L541 (12.8625, 21.4375) -> (12.8625, 25.725)
  line L542 (12.8625, 25.725) -> (17.15, 25.725)
  line L543 (17.15, 25.725) -> (17.15, 21.4375)
  line L544 (12.8625, 21.4375) -> (8.575, 21.4375)
  line L545 (8.575, 21.4375) -> (8.575, 25.725)
  line L546 (8.575, 25.725) -> (12.8625, 25.725)
  line L547 (12.8625, 25.725) -> (12.8625, 21.4375)
  line L548 (8.575, 21.4375) -> (4.2875, 21.4375)
  line L549 (4.2875, 21.4375) -> (4.2875, 25.725)
  line L550 (4.2875, 25.725) -> (8.575, 25.725)
  line L551 (8.575, 25.725) -> (8.575, 21.4375)
  line L552 (4.2875, 21.4375) -> (0, 21.4375)
  line L553 (0, 21.4375) -> (0, 25.725)
  line L554 (0, 25.725) -> (4.2875, 25.725)
  line L555 (4.2875, 25.725) -> (4.2875, 21.4375)
  line L556 (0, 21.4375) -> (-4.2875, 21.4375)
  line L557 (-4.2875, 21.4375) -> (-4.2875, 25.725)
  line L558 (-4.2875, 25.725) -> (0, 25.725)
  line L559 (0, 25.725) -> (0, 21.4375)
  line L560 (-4.2875, 21.4375) -> (-8.575, 21.4375)
  line L561 (-8.575, 21.4375) -> (-8.575, 25.725)
  line L562 (-8.575, 25.725) -> (-4.2875, 25.725)
  line L563 (-4.2875, 25.725) -> (-4.2875, 21.4375)
  line L564 (-8.575, 21.4375) -> (-12.8625, 21.4375)
  line L565 (-12.8625, 21.4375) -> (-12.8625, 25.725)
  line L566 (-12.8625, 25.725) -> (-8.575, 25.725)
  line L567 (-8.575, 25.725) -> (-8.575, 21.4375)
  line L568 (-12.8625, 21.4375) -> (-17.15, 21.4375)
  line L569 (-17.15, 21.4375) -> (-17.15, 25.725)
  line L570 (-17.15, 25.725) -> (-12.8625, 25.725)
  line L571 (-12.8625, 25.725) -> (-12.8625, 21.4375)
  line L572 (-17.15, 21.4375) -> (-21.4375, 21.4375)
  line L573 (-21.4375, 21.4375) -> (-21.4375, 25.725)
  line L574 (-21.4375, 25.725) -> (-17.15, 25.725)
  line L575 (-17.15, 25.725) -> (-17.15, 21.4375)
  line L576 (-21.4375, 21.4375) -> (-25.725, 21.4375)
  line L577 (-25.725, 21.4375) -> (-25.725, 25.725)
  line L578 (-25.725, 25.725) -> (-21.4375, 25.725)
  line L579 (-21.4375, 25.725) -> (-21.4375, 21.4375)
  point P0 (0, 0)
  dimension "d45" = 51.45
  dimension "d46" = 51.45
  dimension "d51" = 4.2875
  dimension "d54" = 4.2875
  constraints: 1160 end point, 1 horizontal, 1 vertical, 1144 other
  measures "d45" distance of L2.end L1.end
  measures "d46" distance of L1.end L0.end
  measures "d51" distance of L2.end L8.start
  measures "d54" distance of L2.end L52.start
extrude "Segment_1" add sketch "brick_sketch_0.1mm tolerance" along normal blind 2 contours L22 L23 L26 L25 L24 L21
extrude "Segment_2" add sketch "brick_sketch_0.1mm tolerance" along normal blind 2 separate body contours L39 L40 L41 L42
extrude "Segment_3" add sketch "brick_sketch_0.1mm tolerance" along normal blind 2 separate body contours L1 L2 L3 L12
extrude "Segment_4" add sketch "brick_sketch_0.1mm tolerance" along normal blind 2 separate body contours L43 L44 L45 L46 L47 L48 L49 L50 L51 L53 L52 L54 L56 L55
extrude "Segment_5" add sketch "brick_sketch_0.1mm tolerance" along normal blind 2 separate body contours L13 L14 L15 L16 L17 L18 L19 L20
extrude "Segment_6" add sketch "brick_sketch_0.1mm tolerance" along normal blind 2 separate body contours L4 L5 L6 L7 L8 L9 L10 L11
extrude "Segment_7" add sketch "brick_sketch_0.1mm tolerance" along normal blind 2 separate body contours L29 L28 L36 L37 L38 L35 L34 L33 L31 L30 L32 L27
